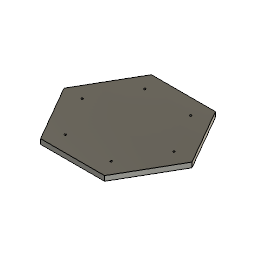
robostus_spyder_body (Autodesk Fusion 360 design; units mm, degrees)
part number: 2025-12-09-12-13-01-708
Autodesk Fusion 360 part; units mm, degrees
sketch "Sketch1" plane through (0, 0, 0) normal (0, 0, 1) x (1, 0, 0)
  line L0 (44.7446, 77.5) -> (-44.7446, 77.5)
  line L1 (-44.7446, 77.5) -> (-89.4893, 0)
  line L2 (-89.4893, 0) -> (-44.7446, -77.5)
  line L3 (-44.7446, -77.5) -> (44.7446, -77.5)
  line L4 (44.7446, -77.5) -> (89.4893, 0)
  line L5 (89.4893, 0) -> (44.7446, 77.5)
  dimension "d1" = 77.5
  measures "d1" distance of origin L5
extrude "Extrude1" add sketch "Sketch1" along normal blind 7
sketch "Sketch2" plane through (0, 0, 7) normal (0, 0, 1) x (-1, 0, 0)
  line L0 (-89.4893, 0) -> (-44.7446, -77.5)
  line L1 (-44.7446, -77.5) -> (44.7446, -77.5)
  line L2 (44.7446, -77.5) -> (89.4893, 0)
  line L3 (89.4893, 0) -> (44.7446, 77.5)
  line L4 (44.7446, 77.5) -> (-44.7446, 77.5)
  line L5 (-44.7446, 77.5) -> (-89.4893, 0)
  line L6 (-32.0429, -77.5) -> (-32.0429, -55.5) construction
  line L7 (-51.0955, -66.5) -> (-32.0429, -55.5) construction
  line L8 (51.0955, -66.5) -> (32.0429, -55.5) construction
  line L9 (32.0429, -77.5) -> (32.0429, -55.5) construction
  line L10 (-83.1384, -11) -> (-64.0859, 0) construction
  line L11 (-83.1384, 11) -> (-64.0859, 0) construction
  line L12 (-32.0429, -77.5) -> (-32.0429, -55.5) construction
  line L13 (-51.0955, -66.5) -> (-32.0429, -55.5) construction
  line L14 (83.1384, 11) -> (64.0859, 0) construction
  line L15 (83.1384, -11) -> (64.0859, 0) construction
  line L16 (32.0429, 77.5) -> (32.0429, 55.5) construction
  line L17 (51.0955, 66.5) -> (32.0429, 55.5) construction
  line L18 (83.1384, 11) -> (64.0859, 0) construction
  line L19 (83.1384, -11) -> (64.0859, 0) construction
  line L20 (-51.0955, 66.5) -> (-32.0429, 55.5) construction
  line L21 (-32.0429, 77.5) -> (-32.0429, 55.5) construction
  circle A0 centre (-32.0429, 55.5) radius 1.5
  circle A1 centre (-64.0859, 0) radius 1.5
  circle A2 centre (-32.0429, -55.5) radius 1.5
  circle A3 centre (32.0429, -55.5) radius 1.5
  circle A4 centre (64.0859, 0) radius 1.5
  circle A5 centre (32.0429, 55.5) radius 1.5
  dimension "d4" = 22
  dimension "d5" = 22
  dimension "d6" = 22
  dimension "d7" = 22
  dimension "d8" = 22
  dimension "d9" = 22
  dimension "d10" = 22
  dimension "d11" = 22
  dimension "d12" = 22
  dimension "d13" = 22
  dimension "d14" = 22
  dimension "d15" = 22
  dimension "d16" = 22
  dimension "d17" = 22
  dimension "d18" = 22
  dimension "d19" = 22
  dimension "d20" = 3
  dimension "d21" = 3
  dimension "d22" = 3
  dimension "d23" = 3
  dimension "d24" = 3
  dimension "d25" = 3
  constraint coincident L1 L6.start
  constraint perpendicular L1 L6
  constraint coincident L0 L7.start
  constraint perpendicular L0 L7
  constraint coincident L6.end L7.end
  constraint coincident L8.end L9.end
  constraint coincident L2 L8.start
  constraint coincident L1 L9.start
  constraint coincident L10.end L11.end
  constraint coincident L0 L10.start
  constraint coincident L5 L11.start
  constraint coincident L14.end L15.end
  constraint coincident L3 L14.start
  constraint coincident L2 L15.start
  constraint perpendicular L3 L14
  constraint perpendicular L2 L15
  constraint perpendicular L5 L11
  constraint perpendicular L0 L10
  constraint perpendicular L2 L8
  constraint perpendicular L1 L9
  constraint coincident L16.end L17.end
  constraint coincident L4 L16.start
  constraint perpendicular L4 L16
  constraint coincident L3 L17.start
  constraint perpendicular L3 L17
  constraint coincident L20.end L21.end
  constraint coincident L4 L21.start
  constraint coincident L5 L20.start
  constraint perpendicular L4 L21
  constraint perpendicular L5 L20
  measures "d4" distance of L6.start L6.end
  measures "d5" distance of L7.start L6.end
  measures "d6" distance of L8.start L8.end
  measures "d7" distance of L9.start L8.end
  measures "d8" distance of L10.start L10.end
  measures "d9" distance of L11.start L10.end
  measures "d10" distance of L6.start L6.end
  measures "d11" distance of L7.start L6.end
  measures "d12" distance of L14.start L14.end
  measures "d13" distance of L15.start L14.end
  measures "d14" distance of L16.end L16.start
  measures "d15" distance of L17.start L16.end
  measures "d16" distance of L14.end L14.start
  measures "d17" distance of L15.start L14.end
  measures "d18" distance of L20.end L20.start
  measures "d19" distance of L21.start L20.end
  measures "d20" diameter of A0
  measures "d21" diameter of A1
  measures "d22" diameter of A2
  measures "d23" diameter of A3
  measures "d24" diameter of A4
  measures "d25" diameter of A5
hole "Hole1" at (32.0429, 55.5, 7) at (64.0859, 0, 7) at (32.0429, -55.5, 7) at (-32.0429, -55.5, 7) at (-32.0429, 55.5, 7) at (-64.0859, 0, 7) direction (0, 0, -1) diameter 2.529 end through all
